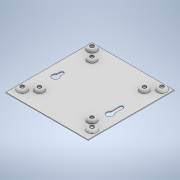
# Autodesk Inventor part: NUC_mount
Saved by Autodesk Inventor 2020 (Build 240168000, 168)
## iProperties
Created: 2019-07-08
Part Number: NUC_mount
Material: Generic
Document SubType Name: Modeling
Designer: Senior Design
Density: 1 g/cm^3
Appearance: Default
Author: Senior Design
Autodesk Inventor part; units mm, degrees
ref_plane "YZ Plane" through (0, 0, 0) normal (1, 0, 0) x (0, 1, 0)
ref_plane "XZ Plane" through (0, 0, 0) normal (0, 1, 0) x (-1, 0, 0)
ref_plane "XY Plane" through (0, 0, 0) normal (0, 0, 1) x (1, 0, 0)
sketch "Sketch1" plane through (0, 0, 0) normal (0, 1, 0) x (-1, 0, 0)
  line L0 (-58.25, -60.95) -> (58.25, -60.95)
  line L1 (58.25, -60.95) -> (58.25, 60.95)
  line L2 (58.25, 60.95) -> (-58.25, 60.95)
  line L3 (-58.25, 60.95) -> (-58.25, -60.95)
  line L4 (-58.25, -60.95) -> (58.25, 60.95) construction
  line L5 (58.25, -60.95) -> (-58.25, 60.95) construction
  point P0 (0, 0)
  dimension "d0" = 121.9
  dimension "d1" = 116.5
  constraints: 12 end point, 2 midpoint, 2 parallel, 1 horizontal, 1 perpendicular
  measures "d0" distance of L0.end L1.end
  measures "d1" distance of L1.end L2.end
extrude "Extrusion1" add sketch "Sketch1" along normal blind 1
sketch "Sketch2" plane through (0, 1, 0) normal (0, 1, 0) x (1, 0, 0)
  circle A0 centre (-49.85, 52.85) radius 6.6
  line L0 (-58.25, -60.95) -> (58.25, -60.95) projected
  line L1 (-58.25, 60.95) -> (-58.25, -60.95) projected
  line L2 (58.25, 60.95) -> (-58.25, 60.95) projected
  circle A1 centre (49.15, 52.85) radius 6.6
  circle A2 centre (-49.85, -46.15) radius 6.6
  circle A3 centre (49.15, -46.15) radius 6.6
  point P0 (0, 0)
  dimension "d5" = 13.2
  dimension "d8" = 8.4
  dimension "d127" = 8.1
  dimension "d130" = 99
  dimension "d133" = 99
  constraints: 4 centre point, 1 horizontal, 1 vertical, 6 other
  measures "d5" diameter of A0
  measures "d8" distance from line of L1 A0.centre
  measures "d127" distance from line of L2 A0.centre
  measures "d130" distance of A0.centre A1.centre
  measures "d133" distance of A0.centre A2.centre
extrude "Extrusion2" cut sketch "Sketch2" against normal through all
sketch "Sketch3" plane through (0, 1, 0) normal (0, 1, 0) x (1, 0, 0)
  circle A0 centre (-37.25, 39.95) radius 6.25
  circle A1 centre (-49.85, 46.15) radius 6.6 projected
  line L0 (-58.25, 60.95) -> (-58.25, -60.95) projected
  line L1 (58.25, 60.95) -> (-58.25, 60.95) projected
  circle A2 centre (37.25, 39.95) radius 6.25
  circle A3 centre (-37.25, -34.55) radius 6.25
  circle A4 centre (37.25, -34.55) radius 6.25
  point P0 (0, 0)
  dimension "d103" = 21
  dimension "d104" = 21
  dimension "d107" = 74.5
  dimension "d110" = 74.5
  constraints: 4 centre point, 1 horizontal, 1 vertical, 6 other
  measures "d103" distance from line of L0 A0.centre
  measures "d104" distance from line of L1 A0.centre
  measures "d107" distance of A0.centre A2.centre
  measures "d110" distance of A0.centre A3.centre
extrude "Extrusion3" cut sketch "Sketch3" against normal blind 1 contours A0 | A2 | A3 | A4
sketch "Sketch4" plane through (0, 1, 0) normal (0, 1, 0) x (1, 0, 0)
  line L0 (-58.25, 60.95) -> (-58.25, -60.95) projected
  line L1 (-58.25, -60.95) -> (58.25, -60.95) projected
  line L2 (58.25, 60.95) -> (-58.25, 60.95) projected
  line L3 (-42.25, -9.05) -> (-39.875, -9.05)
  line L4 (-39.875, -2.5614) -> (-39.875, 2.575)
  line L5 (-39.875, 4.95) -> (-42.25, 4.95)
  line L6 (-44.625, -9.05) -> (-39.875, 4.95) construction
  line L7 (42.25, -16.55) -> (44.625, -16.55)
  line L8 (44.625, -10.0614) -> (44.625, 2.575)
  line L9 (44.625, 4.95) -> (42.25, 4.95)
  line L10 (58.25, -60.95) -> (58.25, 60.95) projected
  arc A0 (-39.875, 2.575) -> (-44.625, 2.575) centre (-42.25, 2.575) ccw
  arc A1 (44.625, 2.575) -> (39.875, 2.575) centre (42.25, 2.575) ccw
  arc A2 (39.875, -10.0614) -> (44.625, -10.0614) centre (42.25, -14.175) ccw
  line L11 (-44.625, 2.575) -> (-44.625, -2.5614)
  line L12 (-44.625, -6.675) -> (-44.625, -9.05)
  line L13 (-44.625, 4.95) -> (-41.4381, -4.4431) construction
  line L14 (-40.2475, -7.952) -> (-39.875, -9.05) construction
  arc A3 (-44.625, -2.5614) -> (-39.875, -2.5614) centre (-42.25, -6.675) ccw
  line L15 (39.875, 2.575) -> (39.875, -10.0614)
  point P0 (0, 0)
  point P1 (-42.25, -2.05)
  point P2 (-42.25, 4.95)
  dimension "d116" = 4.75
  dimension "d117" = 16
  dimension "d118" = 56
  dimension "d119" = 14
  dimension "d121" = 13.625
  dimension "d122" = 21.5
  dimension "d124" = 9.5
  constraints: 24 end point, 10 point on circle, 7 tangent, 5 parallel, 4 centre point, 3 perpendicular, 2 vertical, 1 coincident, 1 collinear, 1 horizontal, 1 midpoint, 1 point on line
  measures "d116" distance of L3.end L6.start
  measures "d117" distance from line of L0 point (-42.25, -2.05)
  measures "d118" distance between parallel lines of L2 L5
  measures "d119" distance of L3.end L5.start
  measures "d121" distance between parallel lines of L10 L8
  measures "d122" distance of L7.end L9.start
  measures "d124" diameter of A2
sketch "Sketch6" plane through (0, 1, 0) normal (0, 1, 0) x (1, 0, 0)
  circle A0 centre (-37.25, 39.95) radius 6.25
  line L0 (58.25, 60.95) -> (-58.25, 60.95)
  line L1 (-58.25, 60.95) -> (-58.25, -60.95)
  circle A1 centre (37.25, 39.95) radius 6.25
  circle A2 centre (-37.25, -34.55) radius 6.25
  circle A3 centre (37.25, -34.55) radius 6.25
  circle A4 centre (-37.25, 39.95) radius 2.3
  circle A5 centre (37.25, 39.95) radius 2.3
  circle A6 centre (-37.25, -34.55) radius 2.3
  circle A7 centre (37.25, -34.55) radius 2.3
  circle A8 centre (-37.25, 39.95) radius 6.25 projected
  point P0 (0, 0)
  dimension "d55" = 74.5
  dimension "d58" = 74.5
  dimension "d70" = 4.6
  dimension "d73" = 74.5
  dimension "d76" = 74.5
  constraints: 8 centre point, 8 coincident, 4 end point, 2 horizontal, 2 vertical, 1 concentric, 18 other
  measures "d55" distance of A0.centre A1.centre
  measures "d58" distance of A0.centre A2.centre
  measures "d70" diameter of A4
  measures "d73" distance of A0.centre point (37.25, 39.95)
  measures "d76" distance of A0.centre point (-37.25, -34.55)
extrude "Extrusion7" add sketch "Sketch6" along normal blind 3.75
fillet "Fillet1" radius 3.7 8 edges at (-43.5, 4.75, 34.55) (31, 4.75, 34.55) (31, 4.75, -39.95) (-43.5, 4.75, -39.95) (34.95, 1, -39.95) (-39.55, 1, -39.95) (34.95, 1, 34.55) (-39.55, 1, 34.55)
sketch "Sketch8" plane through (0, 1, 0) normal (0, 1, 0) x (1, 0, 0)
  circle A0 centre (-49.85, 52.85) radius 6.6
  circle A1 centre (-49.85, 52.85) radius 2.3
  line L0 (58.25, 60.95) -> (-58.25, 60.95) projected
  line L1 (-58.25, 60.95) -> (-58.25, -60.95) projected
  circle A2 centre (49.15, 52.85) radius 2.3
  circle A3 centre (-49.85, -46.15) radius 2.3
  circle A4 centre (49.15, -46.15) radius 2.3
  circle A5 centre (-49.85, 52.85) radius 6.6
  circle A6 centre (-49.85, 52.85) radius 6.6 projected
  circle A7 centre (49.15, 52.85) radius 6.6
  circle A8 centre (-49.85, -46.15) radius 6.6
  circle A9 centre (49.15, -46.15) radius 6.6
  point P0 (0, 0)
  point P1 (-49.85, 46.15)
  dimension "d83" = 4.6
  dimension "d88" = 99
  dimension "d91" = 99
  dimension "d136" = 13.2
  dimension "d139" = 99
  dimension "d142" = 99
  constraints: 9 centre point, 2 concentric, 2 horizontal, 2 vertical, 1 coincident, 12 other
  measures "d83" diameter of A1
  measures "d88" distance of A1.centre A2.centre
  measures "d91" distance of A1.centre A3.centre
  measures "d136" diameter of A0
  measures "d139" distance of A0.centre A7.centre
  measures "d142" distance of A0.centre A8.centre
extrude "Extrusion9" add sketch "Sketch8" along normal blind 3.75
fillet "Fillet3" radius 3.7 8 edges at (-56.45, 4.75, -52.85) (-52.15, 1, -52.85) (-52.15, 1, 46.15) (46.85, 1, 46.15) (46.85, 1, -52.85) (-56.45, 4.75, 46.15) (42.55, 4.75, 46.15) (42.55, 4.75, -52.85)
extrude "Extrusion10" cut sketch "Sketch4" against normal through all contours A3 L11 A0 L4 | A2 L15 A1 L8
equation "\"d55\" = d73"
equation "\"d58\" = d76"
equation "\"d73\" = d107"
equation "\"d76\" = d110"
equation "\"d88\" = d130"
equation "\"d91\" = d133"
equation "\"d136\" = d5"
equation "\"d139\" = d88"
equation "\"d142\" = d91"
equation "\"d121\" = d120"
equation "\"d120\" = 13.625"
body "Solid1"
